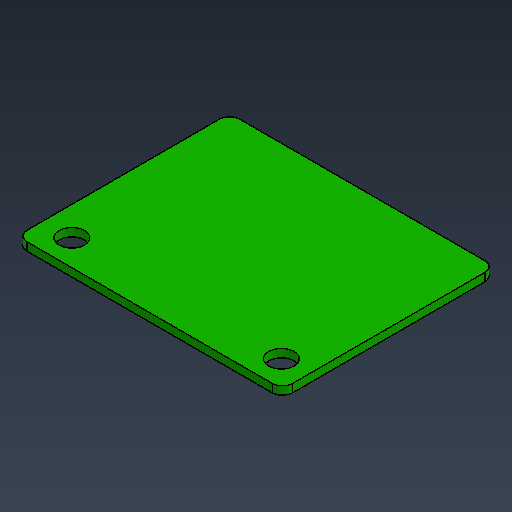
# Autodesk Inventor part: PCB_Motors
Saved by Autodesk Inventor 2026.2 (Build 302298010, 298A)
## iProperties
Created: 2026-04-05
Part Number: PCB_Motors
Material: Generic
Document SubType Name: Modeling
Designer: szymo
Density: 1 g/cm^3
Appearance: Default(1)
Author: szymo
Autodesk Inventor part; units mm, degrees
ref_plane "YZ Plane" through (0, 0, 0) normal (1, 0, 0) x (0, 1, 0)
ref_plane "XZ Plane" through (0, 0, 0) normal (0, 1, 0) x (-1, 0, 0)
ref_plane "XY Plane" through (0, 0, 0) normal (0, 0, 1) x (1, 0, 0)
ref_plane "Work Plane2" through (0.75, 0, 0.1) normal (0, 0, 1) x (1, 0, 0)
sketch "Sketch1" plane through (0.75, 0, 0.1) normal (0, 0, 1) x (1, 0, 0)
  circle A0 centre (15.45, 1.024) radius 2.1 projected
  circle A1 centre (15.45, -5.524) radius 2.1 projected
  line L0 (17.65, 4.2979) -> (17.65, -8.7979) projected
  line L1 (17.65, 4.2979) -> (13.85, 4.2979) projected
  line L2 (14.25, -8.7979) -> (14.25, -8.1479) projected
  line L3 (-17.65, 4.2979) -> (-17.65, -8.7979) projected
  line L4 (-17.65, -8.7979) -> (-13.25, -8.7979) projected
  line L5 (-12.7, -4.4359) -> (-12.7, -5.2359)
  line L6 (11.75, -5.2359) -> (11.75, -4.4359)
  line L7 (13.05, -2.1521) -> (-13.05, -2.1521)
  line L8 (-13.05, -2.1521) -> (-13.05, -1.3521)
  line L9 (-13.05, -1.3521) -> (13.05, -1.3521)
  line L10 (13.05, -1.3521) -> (13.05, -2.1521)
  line L11 (-13.25, 3.6479) -> (-13.25, -8.7979) projected
  circle A2 centre (-15.45, -5.524) radius 2.1 projected
  circle A3 centre (-15.45, 1.024) radius 2.1 projected
  line L12 (-14.25, 3.6479) -> (-13.25, 3.6479) projected
  line L13 (-14.25, 4.2979) -> (-14.25, 3.6479) projected
  line L14 (-17.65, 4.2979) -> (-14.25, 4.2979) projected
  line L15 (17.65, -8.7979) -> (14.25, -8.7979) projected
  line L16 (13.85, 3.6479) -> (13.85, 4.2979) projected
  line L17 (13.85, 3.6479) -> (13.25, 3.6479) projected
  line L18 (13.25, -8.1479) -> (13.25, 3.6479) projected
  line L19 (14.25, -8.1479) -> (13.25, -8.1479) projected
  point P0 (-0.75, 0)
  point P1 (13.65, 3.6479)
  dimension "d5" = 0.8
  dimension "d15" = 0.2
  dimension "d16" = 0.2
  constraints: 12 end point, 3 parallel, 1 horizontal, 1 perpendicular, 1 other
  measures "d5" distance between parallel lines of L7 L9
  measures "d16" distance between parallel lines of L18 L10
extrude "Extrusion1" add sketch "Sketch1" along normal blind 20.9 contours L7 L8 L9 L10
sketch "Sketch2" plane through (-12.3, -2.1521, 0.1) normal (0, -1, 0) x (1, 0, 0)
  line L0 (20.4174, 9.4424) -> (0.5583, 9.4424) construction
  line L1 (0.5583, 9.4424) -> (0.5583, 13.9779) construction
  line L2 (0.5583, 13.9779) -> (20.4174, 13.9779) construction
  line L3 (20.4174, 13.9779) -> (20.4174, 9.4424) construction
  line L4 (17.4954, 12.5546) -> (17.9004, 12.5546)
  line L5 (17.9004, 12.5546) -> (17.9004, 9.929)
  line L6 (17.9004, 9.929) -> (18.6958, 11.7148)
  line L7 (18.6958, 11.7148) -> (18.9428, 11.7148)
  line L8 (18.9428, 11.7148) -> (19.7307, 9.929)
  line L9 (19.7307, 9.929) -> (19.7307, 12.5546)
  line L10 (19.7307, 12.5546) -> (20.1086, 12.5546)
  line L11 (20.1086, 12.5546) -> (20.1086, 9.5066)
  line L12 (20.1086, 9.5066) -> (19.5554, 9.5066)
  line L13 (19.5554, 9.5066) -> (18.7946, 11.2035)
  line L14 (18.7946, 11.2035) -> (18.0585, 9.5066)
  line L15 (18.0585, 9.5066) -> (17.4954, 9.5066)
  line L16 (17.4954, 9.5066) -> (17.4954, 12.5546)
  spline S0 degree 2 poles (14.7215, 9.8549) (14.5486, 10.0575) (14.356, 10.6503) (14.356, 11.0306) knots 0 0 0 1 2 2 2
  spline S1 degree 2 poles (14.356, 11.0306) (14.356, 11.4011) (14.5437, 12.0014) (14.7215, 12.2039) knots 0 0 0 1 2 2 2
  spline S2 degree 2 poles (14.7215, 12.2039) (14.9093, 12.4163) (15.4057, 12.6189) (15.7046, 12.6189) knots 0 0 0 1 2 2 2
  spline S3 degree 2 poles (15.7046, 12.6189) (16.0134, 12.6189) (16.5074, 12.4089) (16.6877, 12.2039) knots 0 0 0 1 2 2 2
  spline S4 degree 2 poles (16.6877, 12.2039) (16.863, 12.0014) (17.0508, 11.4061) (17.0508, 11.0306) knots 0 0 0 1 2 2 2
  spline S5 degree 2 poles (17.0508, 11.0306) (17.0508, 10.6478) (16.8606, 10.0649) (16.6852, 9.8549) knots 0 0 0 1 2 2 2
  spline S6 degree 2 poles (16.6852, 9.8549) (16.5074, 9.6524) (16.0109, 9.4424) (15.7046, 9.4424) knots 0 0 0 1 2 2 2
  spline S7 degree 2 poles (15.7046, 9.4424) (15.3934, 9.4424) (14.8944, 9.6598) (14.7215, 9.8549) knots 0 0 0 1 2 2 2
  spline S8 degree 2 poles (14.7783, 11.0306) (14.7783, 10.7293) (14.9093, 10.2625) (15.0278, 10.1093) knots 0 0 0 1 2 2 2
  spline S9 degree 2 poles (15.0278, 10.1093) (15.1488, 9.9512) (15.4897, 9.7932) (15.7021, 9.7932) knots 0 0 0 1 2 2 2
  spline S10 degree 2 poles (15.7021, 9.7932) (15.922, 9.7932) (16.2529, 9.9463) (16.3789, 10.1093) knots 0 0 0 1 2 2 2
  spline S11 degree 2 poles (16.3789, 10.1093) (16.4999, 10.2649) (16.6284, 10.7342) (16.6284, 11.0306) knots 0 0 0 1 2 2 2
  spline S12 degree 2 poles (16.6284, 11.0306) (16.6284, 11.6309) (16.1245, 12.2681) (15.7021, 12.2681) knots 0 0 0 1 2 2 2
  spline S13 degree 2 poles (15.7021, 12.2681) (15.2798, 12.2681) (14.7783, 11.6309) (14.7783, 11.0306) knots 0 0 0 1 2 2 2
  line L17 (13.2, 12.5546) -> (13.2, 9.8673)
  line L18 (13.2, 9.8673) -> (14.2226, 9.8673)
  line L19 (14.2226, 9.8673) -> (14.2226, 9.5066)
  line L20 (14.2226, 9.5066) -> (11.7723, 9.5066)
  line L21 (11.7723, 9.5066) -> (11.7723, 9.8673)
  line L22 (11.7723, 9.8673) -> (12.7949, 9.8673)
  line L23 (12.7949, 9.8673) -> (12.7949, 12.5546)
  line L24 (12.7949, 12.5546) -> (13.2, 12.5546)
  spline S14 degree 2 poles (9.3073, 9.8549) (9.1344, 10.0575) (8.9417, 10.6503) (8.9417, 11.0306) knots 0 0 0 1 2 2 2
  spline S15 degree 2 poles (8.9417, 11.0306) (8.9417, 11.4011) (9.1294, 12.0014) (9.3073, 12.2039) knots 0 0 0 1 2 2 2
  spline S16 degree 2 poles (9.3073, 12.2039) (9.495, 12.4163) (9.9915, 12.6189) (10.2903, 12.6189) knots 0 0 0 1 2 2 2
  spline S17 degree 2 poles (10.2903, 12.6189) (10.5991, 12.6189) (11.0931, 12.4089) (11.2734, 12.2039) knots 0 0 0 1 2 2 2
  spline S18 degree 2 poles (11.2734, 12.2039) (11.4488, 12.0014) (11.6365, 11.4061) (11.6365, 11.0306) knots 0 0 0 1 2 2 2
  spline S19 degree 2 poles (11.6365, 11.0306) (11.6365, 10.6478) (11.4463, 10.0649) (11.2709, 9.8549) knots 0 0 0 1 2 2 2
  spline S20 degree 2 poles (11.2709, 9.8549) (11.0931, 9.6524) (10.5966, 9.4424) (10.2903, 9.4424) knots 0 0 0 1 2 2 2
  spline S21 degree 2 poles (10.2903, 9.4424) (9.9791, 9.4424) (9.4802, 9.6598) (9.3073, 9.8549) knots 0 0 0 1 2 2 2
  spline S22 degree 2 poles (9.3641, 11.0306) (9.3641, 10.7293) (9.495, 10.2625) (9.6135, 10.1093) knots 0 0 0 1 2 2 2
  spline S23 degree 2 poles (9.6135, 10.1093) (9.7346, 9.9512) (10.0754, 9.7932) (10.2879, 9.7932) knots 0 0 0 1 2 2 2
  spline S24 degree 2 poles (10.2879, 9.7932) (10.5077, 9.7932) (10.8387, 9.9463) (10.9646, 10.1093) knots 0 0 0 1 2 2 2
  spline S25 degree 2 poles (10.9646, 10.1093) (11.0857, 10.2649) (11.2141, 10.7342) (11.2141, 11.0306) knots 0 0 0 1 2 2 2
  spline S26 degree 2 poles (11.2141, 11.0306) (11.2141, 11.6309) (10.7102, 12.2681) (10.2879, 12.2681) knots 0 0 0 1 2 2 2
  spline S27 degree 2 poles (10.2879, 12.2681) (9.8655, 12.2681) (9.3641, 11.6309) (9.3641, 11.0306) knots 0 0 0 1 2 2 2
  line L25 (6.1382, 12.5546) -> (6.6643, 12.5546)
  line L26 (6.6643, 12.5546) -> (7.6277, 11.3419)
  line L27 (7.6277, 11.3419) -> (8.092, 11.3419)
  line L28 (8.092, 11.3419) -> (8.092, 12.5546)
  line L29 (8.092, 12.5546) -> (8.4971, 12.5546)
  line L30 (8.4971, 12.5546) -> (8.4971, 9.5066)
  line L31 (8.4971, 9.5066) -> (7.7116, 9.5066)
  spline S28 degree 2 poles (7.7116, 9.5066) (7.4498, 9.5066) (7.0966, 9.5635) (6.936, 9.6672) knots 0 0 0 1 2 2 2
  spline S29 degree 2 poles (6.936, 9.6672) (6.7755, 9.7709) (6.5902, 10.0945) (6.5902, 10.3341) knots 0 0 0 1 2 2 2
  spline S30 degree 2 poles (6.5902, 10.3341) (6.5902, 10.6676) (6.9311, 11.1196) (7.2226, 11.2282) knots 0 0 0 1 2 2 2
  line L32 (7.2226, 11.2282) -> (6.1382, 12.5546)
  spline S31 degree 2 poles (7.0126, 10.3662) (7.0126, 10.2328) (7.1065, 10.0278) (7.2053, 9.9611) knots 0 0 0 1 2 2 2
  spline S32 degree 2 poles (7.2053, 9.9611) (7.2917, 9.9043) (7.5214, 9.8574) (7.6894, 9.8574) knots 0 0 0 1 2 2 2
  line L33 (7.6894, 9.8574) -> (8.092, 9.8574)
  line L34 (8.092, 9.8574) -> (8.092, 11.0035)
  line L35 (8.092, 11.0035) -> (7.7363, 11.0035)
  spline S33 degree 2 poles (7.7363, 11.0035) (7.561, 11.0035) (7.2818, 10.9417) (7.1855, 10.8454) knots 0 0 0 1 2 2 2
  spline S34 degree 2 poles (7.1855, 10.8454) (7.0966, 10.7614) (7.0126, 10.5243) (7.0126, 10.3662) knots 0 0 0 1 2 2 2
  spline S35 degree 2 poles (5.0465, 12.609) (5.3775, 12.609) (5.8418, 12.4707) (6.0468, 12.3719) knots 0 0 0 1 2 2 2
  line L36 (6.0468, 12.3719) -> (6.0468, 11.863)
  line L37 (6.0468, 11.863) -> (6.0172, 11.863)
  spline S36 degree 2 poles (6.0172, 11.863) (5.8171, 12.0508) (5.3108, 12.2582) (5.0761, 12.2582) knots 0 0 0 1 2 2 2
  spline S37 degree 2 poles (5.0761, 12.2582) (4.7402, 12.2582) (4.3969, 11.9791) (4.3969, 11.7494) knots 0 0 0 1 2 2 2
  spline S38 degree 2 poles (4.3969, 11.7494) (4.3969, 11.5666) (4.5772, 11.3394) (4.7723, 11.2826) knots 0 0 0 1 2 2 2
  spline S39 degree 2 poles (4.7723, 11.2826) (4.9131, 11.2431) (5.1478, 11.1887) (5.3231, 11.1443) knots 0 0 0 1 2 2 2
  spline S40 degree 2 poles (5.3231, 11.1443) (5.4812, 11.1023) (5.7307, 10.9763) (5.827, 10.875) knots 0 0 0 1 2 2 2
  spline S41 degree 2 poles (5.827, 10.875) (5.9209, 10.7738) (6.0246, 10.5021) (6.0246, 10.3242) knots 0 0 0 1 2 2 2
  spline S42 degree 2 poles (6.0246, 10.3242) (6.0246, 9.9537) (5.4466, 9.4523) (4.9996, 9.4523) knots 0 0 0 1 2 2 2
  spline S43 degree 2 poles (4.9996, 9.4523) (4.7427, 9.4523) (4.2882, 9.5536) (4.0931, 9.6499) knots 0 0 0 1 2 2 2
  line L38 (4.0931, 9.6499) -> (4.0931, 10.134)
  line L39 (4.0931, 10.134) -> (4.1227, 10.134)
  spline S44 degree 2 poles (4.1227, 10.134) (4.2684, 10.0006) (4.7229, 9.803) (4.9724, 9.803) knots 0 0 0 1 2 2 2
  spline S45 degree 2 poles (4.9724, 9.803) (5.254, 9.803) (5.6022, 10.0673) (5.6022, 10.2822) knots 0 0 0 1 2 2 2
  spline S46 degree 2 poles (5.6022, 10.2822) (5.6022, 10.4749) (5.3972, 10.7046) (5.2046, 10.7565) knots 0 0 0 1 2 2 2
  spline S47 degree 2 poles (5.2046, 10.7565) (5.0761, 10.7911) (4.7032, 10.88) (4.5797, 10.917) knots 0 0 0 1 2 2 2
  spline S48 degree 2 poles (4.5797, 10.917) (4.266, 11.0134) (3.9745, 11.4011) (3.9745, 11.6852) knots 0 0 0 1 2 2 2
  spline S49 degree 2 poles (3.9745, 11.6852) (3.9745, 11.8655) (4.1202, 12.2113) (4.2511, 12.3323) knots 0 0 0 1 2 2 2
  spline S50 degree 2 poles (4.2511, 12.3323) (4.3969, 12.4657) (4.7674, 12.609) (5.0465, 12.609) knots 0 0 0 1 2 2 2
  point P0 (12.3, -0.1)
  constraints: 2 other
extrude "Extrusion2" cut sketch "Sketch2" against normal blind 0.1
sketch "Sketch3" plane through (-12.3, -2.1521, 0.1) normal (0, -1, 0) x (1, 0, 0)
  arc A0 (20.7, 16.6) -> (21.7, 15.6) centre (21.7, 16.6) ccw projected
  line L0 (20.7, 21.1) -> (20.7, 16.6) projected
  line L1 (26.2, 21.1) -> (20.7, 21.1) projected
  line L2 (26.2, 21.1) -> (26.2, 15.6) projected
  line L3 (21.7, 15.6) -> (26.2, 15.6) projected
  circle A1 centre (23.45, 18.35) radius 1.25 projected
  arc A2 (4.6, 15.6) -> (5.6, 16.6) centre (4.6, 16.6) ccw projected
  line L4 (0.1, 15.6) -> (4.6, 15.6) projected
  line L5 (0.1, 21.1) -> (0.1, 15.6) projected
  line L6 (5.6, 21.1) -> (0.1, 21.1) projected
  line L7 (5.6, 21.1) -> (5.6, 16.6) projected
  circle A3 centre (2.85, 18.35) radius 1.25 projected
  point P0 (12.3, -0.1)
  point P1 (22.45, 18.35)
  point P2 (2.55, 18.35)
hole "Hole1" at (11.15, -2.1521, 18.45) at (-9.45, -2.1521, 18.45) direction (0, 1, 0) diameter 2.5 end through all
fillet "Fillet1" radius 1 4 edges at (13.8, -1.7521, 0.1) (-12.3, -1.7521, 0.1) (-12.3, -1.7521, 21) (13.8, -1.7521, 21)
equation "\"d15\" = d16"
body "Solid1"
